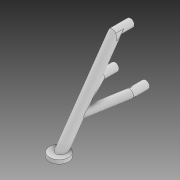
# Autodesk Inventor part: Leg
Saved by Autodesk Inventor 2020 (Build 240168000, 168)
## iProperties
Created: 2021-03-26
Part Number: Leg
Material: Generic
Document SubType Name: Modeling
Designer: DDeGo
Density: 1 g/cm^3
Appearance: Default
Author: DDeGo
Autodesk Inventor part; units mm, degrees
ref_plane "YZ Plane" through (0, 0, 0) normal (1, 0, 0) x (0, 1, 0)
ref_plane "XY Plane" through (0, 0, 0) normal (0, 0, 1) x (1, 0, 0)
sketch "Sketch1" plane through (0, 0, 0) normal (0, 0, 1) x (1, 0, 0)
  line L0 (-4, -6) -> (4, -6) construction
  line L1 (4, -6) -> (4, 6) construction
  line L2 (4, 6) -> (-4, 6) construction
  line L3 (-4, 6) -> (-4, -6) construction
  line L4 (-4, -6) -> (4, 6) construction
  line L5 (4, -6) -> (-4, 6) construction
  circle A0 centre (0, 6) radius 1
  circle A1 centre (-4, -6) radius 1
  circle A2 centre (4, -6) radius 1
  point P0 (0, 0)
  dimension "d0" = 8
  dimension "d1" = 12
  dimension "d2" = 2
  constraints: 12 end point, 3 centre point, 3 midpoint, 2 coincident, 2 equal radius, 2 parallel, 1 horizontal, 1 perpendicular
  measures "d0" distance of L0.start L0.end
  measures "d1" distance of L0.end L1.end
  measures "d2" diameter of A0
extrude "Extrusion1" add sketch "Sketch1" along normal blind 4
sketch "Sketch3" plane through (0, 0, 0) normal (1, 0, 0) x (0, 1, 0)
  line L0 (7, 4) -> (5, 4)
  line L1 (6, 4) -> (-15, 18.704358)
  point P0 (0, 0)
  point P1 (-8, 13.802906)
  dimension "d5" = 35
  dimension "d6" = 15
  dimension "d19" = 8
  constraints: 2 end point, 1 midpoint, 1 point on line
  measures "d5" angle of L1 L0
  measures "d6" horizontal distance of point (0, 0) L1.end
  measures "d19" horizontal distance of point (0, 0) point (-8, 13.803)
ref_plane "Work Plane1" through (0, -15, 18.704358) normal (0, -0.819152, 0.5735764) x (1, 0, 0)
sketch "Sketch4" plane through (0, -15, 18.704358) normal (0, -0.819152, 0.5735764) x (1, 0, 0)
  circle A0 centre (0, 0) radius 1.25
  point P0 (0, -6.718067)
  point P1 (0, 0)
  dimension "d7" = 2.5
  constraints: 1 centre point, 1 coincident
  measures "d7" diameter of A0
extrude "Extrusion2" add sketch "Sketch4" against normal blind 32.25
sketch "Sketch5" plane through (0, 6, 0) normal (0, 0, -1) x (-1, 0, 0)
  circle A0 centre (0, 0) radius 1
  line L0 (1.25, -21) -> (1.25, 5.417653)
  circle A1 centre (0, 0) radius 1
  arc A2 (1.25, -1.198958) -> (0.916667, 0.399653) centre (-2.75, -1.198958) ccw
  line L1 (-1.25, -21) -> (-1.25, 5.417653)
  arc A3 (-0.916667, 0.399653) -> (-1.25, -1.198958) centre (2.75, -1.198958) ccw
  line L2 (1.25, -1.198958) -> (-1.25, -1.198958) construction
  line L3 (-1.25, -1.198958) -> (-1.25, 8.763642)
  line L4 (-1.25, 8.763642) -> (1.25, 8.763642)
  line L5 (1.25, 8.763642) -> (1.25, -1.198958)
  point P0 (0, -6)
  point P1 (-0.916667, 0.399653)
  point P2 (0.916667, 0.399653)
  dimension "d10" = 4
  constraints: 8 end point, 6 point on circle, 4 tangent, 2 centre point, 2 parallel, 2 point on line, 1 equal radius, 1 horizontal, 1 perpendicular
  measures "d10" radius of A2
extrude "Extrusion3" cut sketch "Sketch5" against normal through all both and the other way through all contours A0 A3 L1 L3 L4 L5 L0 A2
ref_plane "Work Plane2" through (0, -15, 18.704358) normal (0, 1, 0) x (-1, 0, 0)
sketch "Sketch6" plane through (0, -15, 18.704358) normal (0, 1, 0) x (-1, 0, 0)
  ellipse E0 centre (0, 0) end of major axis (-1.25, 0) minor radius 1.02394
  circle A0 centre (0, 0) radius 2.5
  point P0 (0, -18.704358)
  dimension "d13" = 5
  constraints: 1 centre point, 1 coincident, 1 other
  measures "d13" diameter of A0
extrude "Extrusion4" add sketch "Sketch6" along normal mid plane 2 contours E0 | A0
sketch "Sketch7" plane through (0, -16, 18.704358) normal (0, -1, 0) x (1, 0, 0)
  circle A0 centre (0, 0) radius 2.5 projected
  point P0 (0, -18.704358)
extrude "Extrusion5" cut sketch "Sketch7" against normal blind 1
sketch "Sketch8" plane through (-4, -6, 4) normal (0, 0, 1) x (1, 0, 0)
  circle A0 centre (0, 0) radius 1 projected
  point P0 (4, 6)
  constraints: 1 coincident
ref_plane "Work Plane3" through (-4, -6, 4) normal (0.3712356, -0.1856178, 0.9097968) x (0.4472136, 0.8944272, 0)
sketch "Sketch9" plane through (-4, -6, 4) normal (0.3712356, -0.1856178, 0.9097968) x (0.4472136, 0.8944272, 0)
  circle A0 centre (0, 0) radius 1
  point P0 (7.155418, -2.473963)
  dimension "d20" = 2
  constraints: 1 centre point, 1 coincident
  measures "d20" diameter of A0
extrude "Extrusion6" add sketch "Sketch9" along normal blind 11 and the other way blind 0.75
sketch "Sketch10" plane through (-4, -6, 0) normal (0, 0, -1) x (-1, 0, 0)
  arc A0 (0.587021, -0.809571) -> (-0.295444, 0.95536) centre (0, 0) ccw
  ellipse E0 centre (0.278427, 0.139213) end of major axis (-0.168787, 1.033641) minor radius 0.909797 (0.587021, -0.809571) -> (-0.295444, 0.95536) ccw
  point P0 (-4, 6)
  constraints: 1 other
extrude "Extrusion7" cut sketch "Sketch10" against normal blind 11
mirror "Mirror1" about plane through (0, 0, 0) normal (1, 0, 0) of "Extrusion7", "Extrusion6"
body "Solid1"
